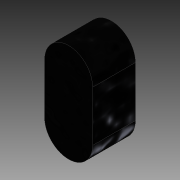
# Autodesk Inventor part: Dopje
Saved by Autodesk Inventor 2015 (Build 190159000, 159)
## iProperties
Created: 2016-01-04
Part Number: Dopje
Material: Generic
Document SubType Name: Modeling
Designer: david
Density: 1 g/cm^3
Appearance: Black
Author: david
Autodesk Inventor part; units mm, degrees
ref_plane "YZ Plane" through (0, 0, 0) normal (1, 0, 0) x (0, 1, 0)
ref_plane "XZ Plane" through (0, 0, 0) normal (0, 1, 0) x (-1, 0, 0)
ref_plane "XY Plane" through (0, 0, 0) normal (0, 0, 1) x (1, 0, 0)
sketch "Sketch1" plane through (0, 0, 0) normal (0, 1, 0) x (-1, 0, 0)
  line L0 (0, 0) -> (0, -23.5) construction
  line L1 (-11.25, 0) -> (-11.25, -23.5)
  line L2 (11.25, -23.5) -> (11.25, 0)
  arc A0 (11.25, 0) -> (-11.25, 0) centre (0, 0) ccw
  arc A1 (-11.25, -23.5) -> (11.25, -23.5) centre (0, -23.5) ccw
  point P0 (0, -11.75)
  dimension "d0" = 23.5
  dimension "d1" = 22.5
  constraints: 8 end point, 4 point on circle, 4 tangent, 2 centre point, 1 midpoint, 1 parallel, 1 vertical
  measures "d0" distance of L0.start L0.end
  measures "d1" diameter of A1
extrude "Extrusion1" add sketch "Sketch1" along normal blind 1
sketch "Sketch2" plane through (0, 1, 0) normal (0, 1, 0) x (1, 0, 0)
  arc A0 (11.25, 23.5) -> (-11.25, 23.5) centre (0, 23.5) ccw projected
  line L0 (0, 0) -> (0, 23.5) construction
  line L1 (11.25, 0) -> (11.25, 23.5)
  line L2 (-11.25, 23.5) -> (-11.25, 0)
  arc A1 (-11.25, 0) -> (11.25, 0) centre (0, 0) ccw
  arc A2 (11.25, 23.5) -> (-11.25, 23.5) centre (0, 23.5) ccw
  line L3 (0, 0) -> (0, 23.5) construction
  line L4 (10, 0) -> (10, 23.5)
  line L5 (-10, 23.5) -> (-10, 0)
  arc A3 (-10, 0) -> (10, 0) centre (0, 0) ccw
  arc A4 (10, 23.5) -> (-10, 23.5) centre (0, 23.5) ccw
  point P0 (0, 11.75)
  point P1 (0, 11.75)
  dimension "d4" = 20
  constraints: 16 end point, 8 point on circle, 8 tangent, 4 centre point, 3 equal length, 2 midpoint, 1 vertical
  measures "d4" diameter of A4
extrude "Extrusion2" add sketch "Sketch2" along normal blind 19
body "Solid1"
